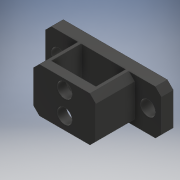
# Autodesk Inventor part: WA03
Saved by Autodesk Inventor 2017 (Build 210142000, 142)
## iProperties
Created: 2019-05-07
Part Number: WA03
Material: ABS Plastic
Document SubType Name: Modeling
Designer: Dell
Density: 1.06 g/cm^3
Appearance: Smooth - Black
Author: Dell
Autodesk Inventor part; units mm, degrees
ref_plane "YZ Plane" through (0, 0, 0) normal (1, 0, 0) x (0, 1, 0)
ref_plane "XZ Plane" through (0, 0, 0) normal (0, 1, 0) x (-1, 0, 0)
ref_plane "XY Plane" through (0, 0, 0) normal (0, 0, 1) x (1, 0, 0)
sketch "Sketch4" plane through (0, 0, 0) normal (0, 0, 1) x (1, 0, 0)
  line L0 (0, 0) -> (12, 0)
  line L1 (12, 0) -> (12, -10)
  line L2 (12, -10) -> (27, -10)
  line L3 (27, -10) -> (27, 0)
  line L4 (27, 0) -> (39, 0)
  line L5 (0, -3) -> (9, -3)
  line L6 (9, -3) -> (9, -13)
  line L7 (9, -13) -> (30, -13)
  line L8 (30, -13) -> (30, -3)
  line L9 (30, -3) -> (39, -3)
  line L10 (0, -3) -> (0, 0)
  line L11 (39, -3) -> (39, 0)
  dimension "d14" = 12
  dimension "d15" = 12
  dimension "d16" = 10
  dimension "d17" = 15
  dimension "d18" = 3
  constraints: 24 end point, 6 perpendicular, 2 point on line, 2 vertical, 1 horizontal, 4 other
  measures "d14" distance of L0.start L0.end
  measures "d15" distance of L3.end L4.end
  measures "d16" distance of L0.end L1.end
  measures "d17" distance of L1.end L2.end
  measures "d18" distance between parallel lines of L0 L5
extrude "Extrusion4" add sketch "Sketch4" along normal blind 30
sketch "Sketch5" plane through (0, 0, 0) normal (0, 1, 0) x (1, 0, 0)
  line L0 (9, 0) -> (0, 0) construction
  line L1 (9, 0) -> (9, -30) construction
  line L2 (0, -30) -> (9, -30) construction
  line L3 (0, 0) -> (0, -30) construction
  line L4 (39, 0) -> (30, 0) construction
  line L5 (39, 0) -> (39, -30) construction
  line L6 (30, -30) -> (39, -30) construction
  line L7 (30, 0) -> (30, -30) construction
  circle A0 centre (4.5, -22.5) radius 2.5
  circle A1 centre (4.5, -7.5) radius 2.5
  line L8 (4.5, -22.5) -> (4.5, -7.5) construction
  line L9 (19.5, -30) -> (19.5, 0)
  line L10 (12, 0) -> (27, 0) projected
  line L11 (27, -30) -> (12, -30) projected
  circle A2 centre (34.5, -22.5) radius 2.5
  circle A3 centre (34.5, -7.5) radius 2.5
  line L12 (34.5, -22.5) -> (34.5, -7.5) construction
  point P0 (4.5, -30)
  point P1 (4.5, 0)
  point P2 (4.5, -15)
  point P3 (0, -15)
  point P4 (34.5, -15)
  dimension "d21" = 5
  dimension "d22" = 5
  dimension "d23" = 15
  constraints: 10 end point, 6 midpoint, 4 centre point, 3 symmetric about line, 2 vertical alignment, 1 horizontal alignment, 1 vertical, 2 other
  measures "d21" diameter of A0
  measures "d22" diameter of A1
  measures "d23" distance of L8.end L8.start
extrude "Extrusion5" cut sketch "Sketch5" against normal through all
sketch "Sketch6" plane through (9, -13, 0) normal (0, -1, 0) x (1, 0, 0)
  line L0 (3, 30) -> (-9, 30) projected
  line L1 (30, 0) -> (30, 30) projected
  line L2 (-9, 30) -> (30, 30)
  line L3 (30, 30) -> (30, 15)
  line L4 (30, 15) -> (-9, 15)
  line L5 (-9, 15) -> (-9, 30)
  point P0 (-9, 0)
  constraints: 8 end point, 2 parallel, 1 horizontal, 1 midpoint, 1 perpendicular
extrude "Extrusion6" cut sketch "Sketch6" against normal through all
sketch "Sketch7" plane through (9, -13, 0) normal (0, -1, 0) x (1, 0, 0)
  circle A0 centre (10.5, 11.7) radius 2.5
  circle A1 centre (10.5, 4.2) radius 2.5
  line L0 (10.5, 4.2) -> (10.5, 11.7) construction
  line L1 (21, 15) -> (0, 15) projected
  point P0 (-9, 0)
  point P1 (10.5, 15)
  dimension "d28" = 5
  dimension "d29" = 5
  dimension "d30" = 7.5
  dimension "d31" = 3.3
  constraints: 2 centre point, 2 end point, 1 midpoint, 1 vertical, 1 vertical alignment
  measures "d28" diameter of A0
  measures "d29" diameter of A1
  measures "d30" distance of L0.start L0.end
  measures "d31" distance from line of L1 L0.end
extrude "Extrusion7" cut sketch "Sketch7" against normal through all
sketch "Sketch8" plane through (0, 0, 0) normal (0, 1, 0) x (1, 0, 0)
  line L0 (27, -15) -> (39, -15) projected
  line L1 (0, 0) -> (39, 0)
  line L2 (39, 0) -> (39, -15)
  line L3 (39, -15) -> (0, -15)
  line L4 (0, -15) -> (0, 0)
  circle A0 centre (4.5, -7.5) radius 2.5 projected
  circle A1 centre (34.5, -7.5) radius 2.5 projected
  constraints: 8 end point, 2 parallel, 1 horizontal, 1 perpendicular
extrude "Extrusion8" add sketch "Sketch8" along normal blind 4
sketch "Sketch9" plane through (0, 0, 0) normal (0, -1, 0) x (1, 0, 0)
  line L0 (9, 15) -> (0, 15) projected
  line L1 (0, 0) -> (0, 15) projected
  line L2 (9, 0) -> (0, 0) projected
  line L3 (9, 0) -> (9, 15) projected
  circle A0 centre (4.5, 7.5) radius 2.5 projected
  line L4 (39, 15) -> (30, 15) projected
  line L5 (30, 0) -> (30, 15) projected
  line L6 (39, 0) -> (30, 0) projected
  line L7 (39, 0) -> (39, 15) projected
  circle A1 centre (34.5, 7.5) radius 2.5 projected
extrude "Extrusion9" cut sketch "Sketch9" along normal through all
chamfer "Chamfer1" distance 2 angle 45 4 edges at (9, -6.5, 15) (30, -6.5, 15) (30, -6.5, 0) (9, -6.5, 0)
chamfer "Chamfer2" distance 2 angle 45 4 edges at (39, 2, 15) (39, 2, 0) (0, 2, 0) (0, 2, 15)
equation "\"d15\" = d14"
body "Solid2"
